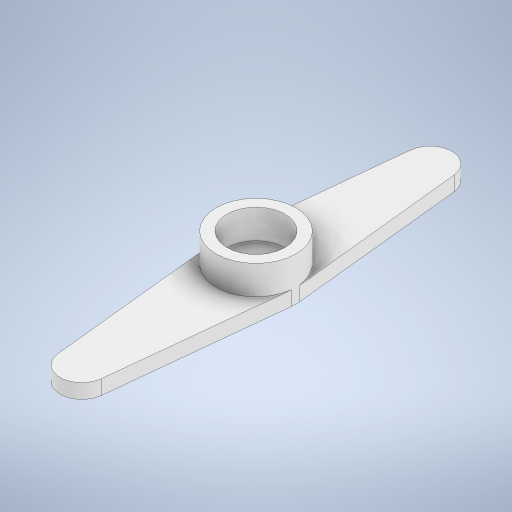
# Autodesk Inventor part: Dual Servo Attachment
Saved by Autodesk Inventor 2024 (Build 280153000, 153)
## iProperties
Created: 2023-04-24
Part Number: Dual Servo Attachment
Material: ABS Plastic
Document SubType Name: Modeling
Designer: byrne
Density: 1.06 g/cm^3
Appearance: Smooth - White
Author: byrne
Autodesk Inventor part; units mm, degrees
ref_plane "YZ Plane" through (0, 0, 0) normal (1, 0, 0) x (0, 1, 0)
ref_plane "XZ Plane" through (0, 0, 0) normal (0, 1, 0) x (-1, 0, 0)
ref_plane "XY Plane" through (0, 0, 0) normal (0, 0, 1) x (1, 0, 0)
sketch "Sketch1" plane through (0, 0, 0) normal (0, 1, 0) x (-1, 0, 0)
  circle A0 centre (0, 0) radius 2.75
  circle A1 centre (0, 12) radius 1.5
  circle A2 centre (0, -12) radius 1.5
  line L0 (0, 12) -> (0, -12) construction
  line L1 (2.735, -0.2865) -> (1.4918, -12.1562)
  line L2 (-1.4918, 12.1563) -> (-2.735, 0.2865)
  line L3 (-1.4918, -12.1562) -> (-2.735, -0.2865)
  line L4 (1.4918, 12.1563) -> (2.735, 0.2865)
  dimension "d0" = 5.5
  dimension "d1" = 3
  dimension "d2" = 27
  constraints: 10 end point, 8 point on circle, 8 tangent, 3 centre point, 2 coincident, 1 equal radius, 1 midpoint, 1 vertical
  measures "d0" diameter of A0
  measures "d1" diameter of A2
extrude "Extrusion1" add sketch "Sketch1" along normal blind 1
sketch "Sketch2" plane through (0, 1, 0) normal (0, 1, 0) x (1, 0, 0)
  circle A0 centre (0, 0) radius 2.75
  circle A1 centre (0, 0) radius 2
  dimension "d5" = 5.5
  dimension "d6" = 4
  constraints: 2 centre point, 2 coincident
  measures "d5" diameter of A0
  measures "d6" diameter of A1
extrude "Extrusion2" add sketch "Sketch2" along normal blind 2
body "Solid1"
